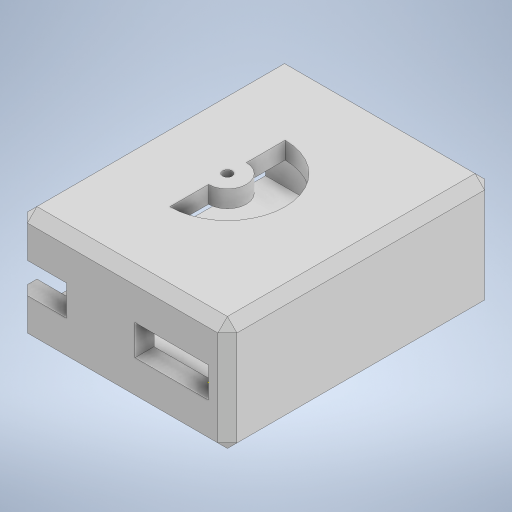
# Autodesk Inventor part: Flywheel Cutting Jig
Saved by Autodesk Inventor 2023 (Build 270158000, 158)
## iProperties
Created: 2022-12-31
Part Number: Flywheel Cutting Jig
Material: Generic
Document SubType Name: Modeling
Designer: tgr41
Density: 1 g/cm^3
Appearance: Default
Author: tgr41
Autodesk Inventor part; units mm, degrees
ref_plane "YZ Plane" through (0, 0, 0) normal (1, 0, 0) x (0, 1, 0)
ref_plane "XZ Plane" through (0, 0, 0) normal (0, 1, 0) x (-1, 0, 0)
ref_plane "XY Plane" through (0, 0, 0) normal (0, 0, 1) x (1, 0, 0)
sketch "Sketch1" plane through (0, 0, 0) normal (0, 1, 0) x (-1, 0, 0)
  line L0 (0, 0) -> (76.2, 0)
  line L1 (76.2, 0) -> (76.2, -76.2)
  line L2 (76.2, -76.2) -> (0, -76.2)
  line L3 (0, -76.2) -> (0, 0)
  line L4 (-6.35, 6.35) -> (76.2, 6.35)
  line L5 (76.2, -82.55) -> (-6.35, -82.55)
  line L6 (-6.35, -82.55) -> (-6.35, 6.35)
  line L7 (76.2, 6.35) -> (63.5, 6.35)
  line L8 (63.5, 6.35) -> (63.5, -82.55)
  line L9 (76.2, -38.1) -> (0, -38.1)
  line L10 (38.1, 0) -> (38.1, -76.2)
  circle A0 centre (38.1, -38.1) radius 3.048
  circle A1 centre (38.1, -38.1) radius 1.5875
  circle A2 centre (38.1, -38.1) radius 6.3171
  circle A3 centre (38.1, -38.1) radius 19.2182
  point P0 (63.5, 0)
  point P1 (63.5, -76.2)
  point P2 (38.1, -57.3182)
  point P3 (38.1, -44.4171)
  point P4 (38.1, -31.7829)
  point P5 (38.1, -18.8818)
  dimension "d0" = 76.2
  dimension "d1" = 76.2
  dimension "d2" = 6.35
  dimension "d3" = 6.35
  dimension "d4" = 6.35
  dimension "d6" = 12.7
  dimension "d7" = 6.096
  dimension "d12" = 3.175
  constraints: 22 end point, 5 midpoint, 4 centre point, 3 coincident, 3 parallel, 2 horizontal, 2 perpendicular, 2 point on line
  measures "d0" distance of L1.end L2.end
  measures "d1" distance of L0.end L1.end
  measures "d2" distance between parallel lines of L5 L2
  measures "d3" distance between parallel lines of L4 L0
  measures "d4" distance between parallel lines of L6 L3
  measures "d6" distance of L4.end L7.end
  measures "d7" diameter of A0
  measures "d12" diameter of A1
extrude "Extrusion1" add sketch "Sketch1" along normal mid plane 38.1 contours L3 L2 L8 L5 L6 L4 L0 | L0 L10 A3 L9 L3 | L0 L8 L9 A3 L10 | L9 A3 L10 L2 L3 | A3 L9 A2 L10 | L10 A2 L9 A3 | L9 A2 L10 A3 | L8 L2 L10 A3 L9 | A2 L9 A0 L10 | L10 A0 L9 A2 | A3 L10 A2 L9 | L9 A0 L10 A2 | A0 L9 A1 L10 | L10 A1 L9 A0 | A2 L10 A0 L9 | L9 A1 L10 A0 | A1 L9 L10 | L10 L9 A1 | A0 L10 A1 L9 | L9 L10 A1 | L9 A1 L10
extrude "Extrusion2" cut sketch "Sketch1" along normal mid plane 26.67 contours L0 L10 A3 L9 L3 | L0 L8 L9 A3 L10 | L9 A3 L10 L2 L3 | A3 L9 A2 L10 | L10 A2 L9 A3 | L9 A2 L10 A3 | L8 L2 L10 A3 L9 | A2 L9 A0 L10 | L10 A0 L9 A2 | A3 L10 A2 L9 | L9 A0 L10 A2 | A0 L9 A1 L10 | L10 A1 L9 A0 | A2 L10 A0 L9 | L9 A1 L10 A0 | A1 L9 L10 | L10 L9 A1 | A0 L10 A1 L9 | L9 L10 A1 | L9 A1 L10
extrude "Extrusion3" cut sketch "Sketch1" along normal blind 26.67 contours A1 L9 L10 | L10 L9 A1 | L9 L10 A1 | L9 A1 L10
extrude "Extrusion4" cut sketch "Sketch1" against normal blind 26.67 contours A0 L9 A1 L10 | L10 A1 L9 A0 | L9 A1 L10 A0 | A1 L9 L10 | L10 L9 A1 | A0 L10 A1 L9 | L9 L10 A1 | L9 A1 L10
extrude "Extrusion5" cut sketch "Sketch1" along normal mid plane 76.2 contours L10 A2 L9 A3 | L9 A2 L10 A3 picked at (24.03, -33.4265) picked at (23.3428, -39.5255)
chamfer "Chamfer1" distance 3.175 angle 45 12 edges at (6.35, -19.05, -38.1) (6.35, 0, -82.55) (6.35, 19.05, -38.1) (6.35, 0, 6.35) (-28.575, -19.05, 6.35) (-28.575, -19.05, -82.55) (-28.575, 19.05, 6.35) (-28.575, 19.05, -82.55) (-63.5, 0, -82.55) (-63.5, 19.05, -38.1) (-63.5, 0, 6.35) (-63.5, -19.05, -38.1)
sketch "Sketch2" plane through (-60.325, 15.875, 6.35) normal (0, 0, 1) x (1, 0, 0)
  line L0 (60.325, -15.875) -> (-14.3464, -15.875)
  line L1 (-14.3464, -15.875) -> (-14.3464, -10.795)
  line L2 (-3.175, -31.75) -> (-3.175, 0) projected
  line L3 (-14.3464, -10.795) -> (60.325, -10.795)
  line L4 (60.325, -29.21) -> (60.325, -2.54) projected
  line L5 (60.325, -10.795) -> (60.325, -20.955)
  line L6 (60.325, -20.955) -> (-14.3464, -20.955)
  line L7 (-14.3464, -20.955) -> (-14.3464, -15.875)
  line L8 (12.9951, -20.955) -> (12.9951, -10.795)
  line L9 (35.8551, -10.795) -> (35.8551, -20.955)
  dimension "d22" = 5.08
  dimension "d23" = 10.16
  dimension "d26" = 24.4699
  dimension "d27" = 22.86
  constraints: 16 end point, 6 point on line, 5 perpendicular, 2 parallel, 1 horizontal
  measures "d22" distance of L0.end L1.end
  measures "d23" distance of L3.end L5.end
  measures "d26" distance between parallel lines of L4 L9
  measures "d27" distance between parallel lines of L9 L8
extrude "Extrusion6" cut sketch "Sketch2" against normal blind 127 contours L4 L6 L9 L0 | L0 L9 L3 L4 | L8 L6 L2 L0 | L0 L2 L3 L8 | L2 L6 L7 L0 | L0 L1 L3 L2
sketch "Sketch3" plane through (-60.325, -15.875, 6.35) normal (0, 0, 1) x (1, 0, 0)
  point P0 (60.325, 15.875)
body "Solid1"
